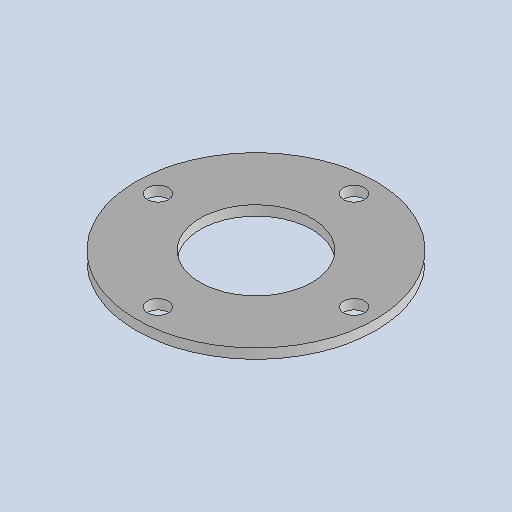
# Autodesk Inventor part: PRS 8133 charging blind flange_940
Saved by Autodesk Inventor 2026.2 (Build 302298000, 298)
## iProperties
Created: 2025-02-13
Part Number: PRS 8133 charging blind flange_940
Material: Steel
Document SubType Name: Sheet Metal
Designer: admin
Mass: 2466.79 g
Surface Area: 934.137 cm^2
Volume: 314.241 cm^3
Density: 7.85 g/cm^3
Flat Pattern Width: 19.5 cm
Flat Pattern Length: 19.5 cm
Flat Pattern Area: 380.25 cm^2
Sheet Metal Rule: AISI304 4mm Die 32
Sheet Metal Width: 195,000 mm
Sheet Metal Length: 195,000 mm
Sheet Metal Area: 38025,000 mm^2
Appearance: Default
Author: pokla
Autodesk Inventor part; units mm, degrees
ref_plane "YZ Plane" through (0, 0, 0) normal (1, 0, 0) x (0, 1, 0)
ref_plane "XZ Plane" through (0, 0, 0) normal (0, 1, 0) x (-1, 0, 0)
ref_plane "XY Plane" through (0, 0, 0) normal (0, 0, 1) x (1, 0, 0)
sketch "Sketch2" plane through (0, 0, 0) normal (0, 0, 1) x (1, 0, 0)
  circle A0 centre (0, 0) radius 45.5
  circle A1 centre (0, 0) radius 97.5
  dimension "d25" = 91
  dimension "d27" = 195
  measures "d25" diameter of A0
  measures "d27" diameter of A1
extrude "Plate2" add sketch "Sketch2" along normal blind 8
sketch "Sketch3" plane through (0, 0, 8) normal (0, 0, 1) x (1, 0, 0)
  circle A0 centre (-80, 0) radius 8.5
  circle A1 centre (0, 0) radius 80 construction
  dimension "d28" = 160
  dimension "d15" = 17
  constraints: 2 horizontal alignment, 1 centre point, 1 coincident, 2 other
  measures "d15" diameter of A0
extrude "Cut1" cut sketch "Sketch3" against normal blind 8
pattern_circular "Circular Pattern1" count 4 over 360 about axis through (0, 0, -10) along (0, 0, 1) of "Cut1"
equation "\"d17\" = Thickness"
equation "\"d14\" = Thickness"
equation "\"BendReliefWidth\" = Thickness"
equation "\"BendReliefDepth\" = 0.5 * Thickness"
equation "\"CornerReliefSize\" = 4 * Thickness"
equation "\"MinimumRemnant\" = 2 * Thickness"
equation "\"TransitionRadius\" = BendRadius"
equation "\"JacobiRadiusSize\" = BendRadius"
equation "\"GapSize\" = Thickness"
equation "\"Thickness\" = 8"
equation "\"BendRadius\" = 6"
body "Solid3"
